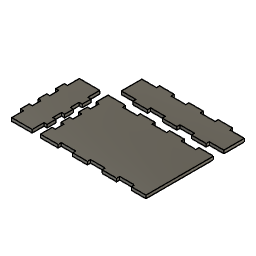
Kartenbox v9 (Autodesk Fusion 360 design; units mm, degrees)
Autodesk Fusion 360 part; units mm, degrees
sketch "Skizze3" plane through (0, 0, 0) normal (0, 0, 1) x (1, 0, 0)
  line L0 (0, 0) -> (103, 0)
  line L1 (103, 0) -> (103, 66)
  line L2 (103, 66) -> (0, 66)
  line L3 (0, 66) -> (0, 0)
  line L4 (-75, 0) -> (-101, 0)
  line L5 (-101, 0) -> (-101, 66)
  line L6 (-101, 66) -> (-75, 66)
  line L7 (-75, 66) -> (-75, 0)
  line L8 (-0.6279, 112.9221) -> (102.3721, 112.9221)
  line L9 (102.3721, 112.9221) -> (102.3721, 138.9221)
  line L10 (102.3721, 138.9221) -> (-0.6279, 138.9221)
  line L11 (-0.6279, 138.9221) -> (-0.6279, 112.9221)
  dimension "d11" = 103
  dimension "d12" = 66
  dimension "d13" = 26
  dimension "d14" = 66
  dimension "d15" = 103
  dimension "d16" = 26
  constraint horizontal L0
  constraint vertical L1
  constraint horizontal L2
  constraint vertical L3
  constraint coincident L0.start L3.end
  constraint horizontal L4
  constraint vertical L5
  constraint horizontal L6
  constraint vertical L7
  constraint horizontal L8
  constraint vertical L9
  constraint horizontal L10
  constraint vertical L11
  measures "d11" distance of L0.start L0.end
  measures "d12" distance of L0.start L2.end
  measures "d13" distance of L4.start L4.end
  measures "d14" distance of L4.start L6.end
  measures "d15" distance of L8.start L8.end
  measures "d16" distance of L8.start L10.end
extrude "Extrusion2" add sketch "Skizze3" along normal blind 3 makes body 1 at (33.7055, 121.5888, 0) makes body 2 at (34.3333, 44, 0) makes body 3 at (-83.6667, 22, 0)
move_body "Verschieben1" bodies 3 to x (1, 0, 0) y (0, 1, 0) z (0, 0, 1) at (70, 0, 0)
move_body "Verschieben2" bodies 1 to x (1, 0, 0) y (0, 1, 0) z (0, 0, 1) at (0, -10, 0)
move_body "Verschieben5" bodies 1 to x (1, 0, 0) y (0, 1, 0) z (0, 0, 1) at (0, -30, 0)
sketch "Skizze8" plane through (0, 0, 3) normal (0, 0, 1) x (-1, 0, 0)
  line L0 (0, -66) -> (0, 0)
  line L1 (0, 0) -> (-103, 0)
  line L2 (-103, 0) -> (-103, -66)
  line L3 (-103, -66) -> (0, -66)
  line L4 (-3, -63) -> (-100, -63)
  line L5 (-100, -63) -> (-100, -3)
  line L6 (-100, -3) -> (-3, -3)
  line L7 (-3, -3) -> (-3, -63)
  line L8 (28, -63) -> (8, -63)
  line L9 (8, -63) -> (8, -3)
  line L10 (8, -3) -> (28, -3)
  line L11 (28, -3) -> (28, -63)
  line L12 (-2.3721, -95.9221) -> (-99.3721, -95.9221)
  line L13 (-99.3721, -95.9221) -> (-99.3721, -75.9221)
  line L14 (-99.3721, -75.9221) -> (-2.3721, -75.9221)
  line L15 (-2.3721, -75.9221) -> (-2.3721, -95.9221)
  line L16 (5, -66) -> (31, -66)
  line L17 (31, -66) -> (31, 0)
  line L18 (31, 0) -> (5, 0)
  line L19 (5, 0) -> (5, -66)
  line L20 (-3, -3) -> (31, -3)
  line L21 (-3, -63) -> (31, -63)
  dimension "d66" = 3
  dimension "d67" = 3
  dimension "d68" = 3
  dimension "d69" = 3
  dimension "d70" = 3
  dimension "d71" = 3
  dimension "d72" = 3
  dimension "d73" = 3
  constraint horizontal L4
  constraint vertical L5
  constraint horizontal L6
  constraint vertical L7
  constraint horizontal L8
  constraint vertical L9
  constraint horizontal L10
  constraint vertical L11
  constraint horizontal L12
  constraint vertical L13
  constraint horizontal L14
  constraint vertical L15
  constraint coincident L17 L20.end
  constraint perpendicular L17 L20
  constraint coincident L17 L21.end
  constraint perpendicular L17 L21
  measures "d66" distance of L2 L5
  measures "d67" distance of L3 L4
  measures "d68" distance of L0 L7
  measures "d69" distance of L1 L6
  measures "d70" distance of L8 L16
  measures "d71" distance of L11 L17
  measures "d72" distance of L9 L19
  measures "d73" distance of L10 L18
move_body "Verschieben6" bodies 1 to x (1, 0, 0) y (0, 1, 0) z (0, 0, 1) at (0.6279, -6.9221, 0)
move_body "Verschieben7" bodies 1 to x (1, 0, 0) y (0, 1, 0) z (0, 0, 1) at (0, 7, 0)
sketch "Skizze10" plane through (0, 0, 3) normal (0, 0, 1) x (-1, 0, 0)
  line L0 (0, -66) -> (0, 0)
  line L1 (0, 0) -> (-103, 0)
  line L2 (-103, 0) -> (-103, -66)
  line L3 (-103, -66) -> (0, -66)
  line L4 (0, -99) -> (0, -73)
  line L5 (0, -73) -> (-103, -73)
  line L6 (-103, -73) -> (-103, -99)
  line L7 (-103, -99) -> (0, -99)
  line L8 (5, -66) -> (31, -66)
  line L9 (31, -66) -> (31, 0)
  line L10 (31, 0) -> (5, 0)
  line L11 (5, 0) -> (5, -66)
  line L12 (28, -3) -> (8, -3)
  line L13 (8, 0) -> (8, -66)
  line L14 (8, -63) -> (28, -63)
  line L15 (28, -66) -> (28, 0)
  line L16 (-3, -3) -> (-100, -3)
  line L17 (-100, -3) -> (-100, -63)
  line L18 (-100, -63) -> (-3, -63)
  line L19 (-3, -63) -> (-3, 0)
  line L20 (0, -76) -> (-103, -76)
  line L21 (-100, -76) -> (-100, -96)
  line L22 (-103, -96) -> (0, -96)
  line L23 (-3, -96) -> (-3, -76)
  line L24 (-3, -63) -> (31, -63)
  line L25 (-3, -63) -> (-3, -99)
  line L26 (-3, -3) -> (31, -3)
  line L27 (-3, -54.4286) -> (31, -54.4286)
  line L28 (-3, -45.8571) -> (31, -45.8571)
  line L29 (-3, -37.2857) -> (31, -37.2857)
  line L30 (-3, -28.7143) -> (31, -28.7143)
  line L31 (-3, -20.1429) -> (31, -20.1429)
  line L32 (-3, -11.5714) -> (31, -11.5714)
  line L33 (-3, -3) -> (31, -3)
  line L34 (-17.2857, -63) -> (-17.2857, -99)
  line L35 (-17.2857, -63) -> (-17.2857, 0)
  line L36 (-31.5714, -63) -> (-31.5714, -99)
  line L37 (-31.5714, -63) -> (-31.5714, 0)
  line L38 (-45.8571, -63) -> (-45.8571, -99)
  line L39 (-45.8571, -63) -> (-45.8571, 0)
  line L40 (-60.1429, -63) -> (-60.1429, -99)
  line L41 (-60.1429, -63) -> (-60.1429, 0)
  line L42 (-74.4286, -63) -> (-74.4286, -99)
  line L43 (-74.4286, -63) -> (-74.4286, 0)
  line L44 (-88.7143, -63) -> (-88.7143, -99)
  line L45 (-88.7143, -63) -> (-88.7143, 0)
  line L46 (-103, -63) -> (-103, -99)
  line L47 (-103, -63) -> (-103, 0)
  dimension "d82" = 0
  dimension "d83" = 60
  dimension "d86" = -100
  dimension "d87" = -100
  constraint coincident L9 L24.end
  constraint perpendicular L9 L24
  constraint coincident L7 L25.end
  constraint perpendicular L7 L25
  constraint coincident L9 L26.end
  constraint perpendicular L9 L26
  constraint coincident L1 L19.end
  constraint coincident L16.start L19
  constraint coincident L23.start L22
  constraint coincident L23.end L20
  constraint coincident L21.start L20
  constraint coincident L21.end L22
  constraint coincident L14.start L13
  constraint coincident L14.end L15
  constraint coincident L12.start L15
  constraint coincident L12.end L13
extrude "Extrusion5" cut sketch "Skizze10" against normal through all contours L0 L19 L27 L28 | L8 L11 L13 L24 | L11 L13 L24 L27 | L3 L18 L34 L36 | L5 L20 L25 L34 | L4 L5 L20 L25 | L4 L20 L22 L23 L25 | L0 L19 L29 L30 | L11 L13 L28 L29 | L1 L16 L35 L37 | L8 L9 L15 L24 | L9 L15 L24 L27 | L3 L18 L38 L40 | L5 L20 L36 L38 | L7 L22 L25 L34 | L4 L7 L22 L25 | L0 L19 L31 L32 | L11 L13 L30 L31 | L9 L15 L28 L29 | L1 L16 L39 L41 | L3 L18 L42 L44 | L5 L20 L40 L42 | L7 L22 L36 L38 | L11 L13 L26 L32 L33 | L10 L11 L13 L26 L33 | L9 L15 L30 L31 | L1 L16 L43 L45 | L5 L6 L20 L44 L46 | L7 L22 L40 L42 | L9 L15 L26 L32 L33 | L9 L10 L15 L26 L33 | L6 L7 L22 L44 L46 bodies 1 2 3
equation "DickeMat = 3 mm"
equation "d11 = 100 mm + DickeMat"
equation "d12 = 60 mm + 2 * DickeMat"
equation "d13 = 20 mm + 2 * DickeMat"
equation "d14 = d12"
equation "d15 = d11"
equation "d16 = 20 mm + 2 * DickeMat"
equation "d17 = DickeMat"
equation "d66 = DickeMat"
equation "d67 = DickeMat"
equation "d68 = DickeMat"
equation "d69 = DickeMat"
equation "d70 = DickeMat"
equation "d71 = DickeMat"
equation "d72 = DickeMat"
equation "d73 = DickeMat"
named bodies: "Seitenplatte", "Vorderseite", "Bodenplatte"
